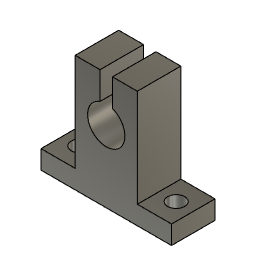
SK 12mm v1 (Autodesk Fusion 360 design; units mm, degrees)
Autodesk Fusion 360 part; units mm, degrees
sketch "Sketch1" plane through (0, 0, 0) normal (0, 1, 0) x (1, 0, 0)
  line L0 (0, 0) -> (42, 0)
  line L1 (0, 0) -> (0, -6)
  line L2 (42, 0) -> (42, -6)
  line L3 (42, -6) -> (31, -6)
  line L4 (31, -6) -> (31, -37.5)
  line L5 (0, -6) -> (11, -6)
  line L6 (11, -6) -> (11, -37.5)
  line L7 (11, -37.5) -> (31, -37.5)
  dimension "d1" = 42
  dimension "d2" = 6
  dimension "d3" = 6
  dimension "d7" = 11
  dimension "d8" = 31.5
  dimension "d9" = 11
  dimension "d10" = 31.5
  constraint coincident L0.start L1.start
  constraint horizontal L0
  constraint perpendicular L0 L1
  constraint perpendicular L0 L2
  constraint perpendicular L2 L3
  constraint perpendicular L3 L4
  constraint perpendicular L1 L5
  constraint perpendicular L5 L6
  measures "d1" distance of L0.start L0.end
  measures "d2" distance of L0.start L1.end L1.start
  measures "d3" distance of L0.end L2.end
  measures "d7" distance of L2.end L3.end
  measures "d8" distance of L3.end L4.end L0.start
  measures "d9" distance of L1.end L5.end
  measures "d10" distance of L5.end L6.end L0.start
extrude "Extrude1" add sketch "Sketch1" along normal blind 14
sketch "Sketch2" plane through (0, 0, 0) normal (0, -1, 0) x (1, 0, 0)
  line L0 (0, 6) -> (0, 0)
  line L1 (0, 0) -> (42, 0)
  line L2 (42, 0) -> (42, 6)
  line L3 (42, 6) -> (31, 6)
  line L4 (31, 6) -> (31, 37.5)
  line L5 (31, 37.5) -> (11, 37.5)
  line L6 (11, 37.5) -> (11, 6)
  line L7 (11, 6) -> (0, 6)
  line L8 (0, 0) -> (21, 0)
  line L9 (21, 0) -> (21, 23)
  circle A0 centre (21, 23) radius 6
  line L10 (21, 37.5) -> (23, 37.5)
  line L11 (21, 37.5) -> (19, 37.5)
  line L12 (19, 37.5) -> (19, 28.6569)
  line L13 (23, 37.5) -> (23, 28.6569)
  dimension "d13" = 23
  dimension "d14" = 12
  dimension "d15" = 2
  dimension "d16" = 2
  constraint coincident L0.end L1.start
  constraint midpoint L1 L8.end
  constraint perpendicular L8 L9
  constraint coincident L9.end A0.centre
  constraint midpoint L5 L10.start
  constraint horizontal L10
  constraint parallel L5 L11
  constraint coincident A0 L12.end
  constraint perpendicular L11 L12
  constraint coincident A0 L13.end
  constraint perpendicular L10 L13
  measures "d13" distance of L8.end L9.end
  measures "d14" diameter of A0
  measures "d15" distance of L10.start L10.end
  measures "d16" distance of L10.start L11.end
extrude "Extrude2" cut sketch "Sketch2" against normal blind 49.568 contours A0 | L5 A0 L10 L11 L12 L13
sketch "Sketch3" plane through (0, 0, 6) normal (0, 0, 1) x (-1, 0, 0)
  line L0 (0, 0) -> (-11, 0)
  line L1 (-11, 0) -> (-11, -14)
  line L2 (-11, -14) -> (0, -14)
  line L3 (0, -14) -> (0, 0)
  line L4 (-5.5, -14) -> (-5.5, 0)
  line L5 (0, -7) -> (-11, -7)
  circle A0 centre (-5.5, -7) radius 2.75
  dimension "d19" = 5.5
  constraint midpoint L2 L4.start
  constraint midpoint L0 L4.end
  constraint midpoint L3 L5.start
  constraint midpoint L1 L5.end
  constraint midpoint L5 A0.centre
  measures "d19" diameter of A0
extrude "Extrude3" cut sketch "Sketch3" against normal blind 15.501 contours L4 L5 A0 | L4 L5 A0 | L4 L5 A0 | L4 L5 A0
sketch "Sketch4" plane through (0, 0, 6) normal (0, 0, 1) x (-1, 0, 0)
  line L0 (-31, 0) -> (-42, 0)
  line L1 (-42, 0) -> (-42, -14)
  line L2 (-42, -14) -> (-31, -14)
  line L3 (-31, -14) -> (-31, 0)
  circle A0 centre (-36.5, -7) radius 2.75
  dimension "d22" = 5.5
  measures "d22" diameter of A0
extrude "Extrude4" cut sketch "Sketch4" against normal blind 36.862 contours A0
